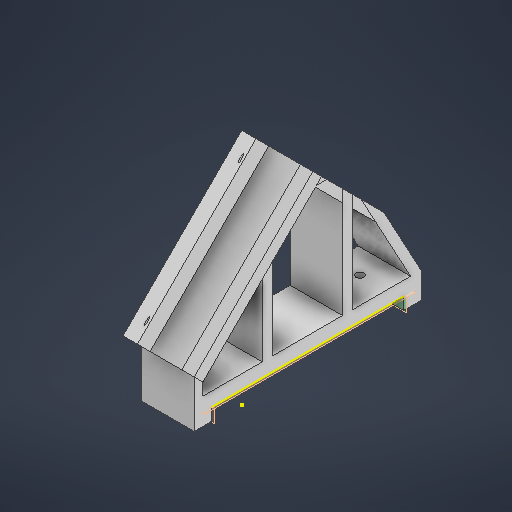
# Autodesk Inventor part: HalterungIso
Saved by Autodesk Inventor 2026.2 (Build 302298000, 298)
## iProperties
Created: 2025-12-13
Part Number: HalterungIso
Material: Generisch
Document SubType Name: Modeling
Designer: alexa
Density: 1 g/cm^3
Appearance: Vorgabe
Author: alexa
Autodesk Inventor part; units mm, degrees
ref_plane "YZ Plane" through (0, 0, 0) normal (1, 0, 0) x (0, 1, 0)
ref_plane "XZ Plane" through (0, 0, 0) normal (0, 1, 0) x (-1, 0, 0)
ref_plane "XY Plane" through (0, 0, 0) normal (0, 0, 1) x (1, 0, 0)
ref_plane "Arbeitsebene1" through (0, 0, 0) normal (0, 0, 1) x (1, 0, 0)
sketch "Skizze1" plane through (0, 0, 0) normal (0, 0, 1) x (1, 0, 0)
  line L0 (15, 55) -> (-15, 55) projected
  line L1 (-15, 55) -> (-15, -55) projected
  line L2 (-15, -55) -> (15, -55) projected
  line L3 (15, -55) -> (15, 55) projected
  circle A0 centre (0, 45) radius 5 projected
  circle A1 centre (0, -45) radius 5 projected
  line L4 (15, 55) -> (-15, 55) projected
  line L5 (-15, 55) -> (-15, -55) projected
  line L6 (-15, -55) -> (15, -55) projected
  line L7 (15, -55) -> (15, 55) projected
  circle A2 centre (0, 45) radius 5 projected
  circle A3 centre (0, -45) radius 5 projected
  point P0 (0, 0)
ref_plane "Arbeitsebene2" through (0, -55, -5) normal (0, -1, 0) x (-1, 0, 0)
sketch "Skizze2" plane through (0, -55, -5) normal (0, -1, 0) x (-1, 0, 0)
  line L0 (15, 2) -> (-15, 2) projected
  line L1 (-15, 2) -> (-15, -2) projected
  line L2 (-15, -2) -> (-15, -5) projected
  line L3 (15, -5) -> (-15, -5) projected
  line L4 (15, 2) -> (15, -5) projected
  point P0 (0, -5)
extrude "Extrusion1" add sketch "Skizze2" along normal blind 10
sketch "Skizze3" plane through (-15, -55, 0) normal (0, 0, 1) x (1, 0, 0)
  line L0 (0, -10) -> (30, -10) projected
  line L1 (30, 0) -> (30, -10) projected
  line L2 (0, -10) -> (30, -10)
  line L3 (30, -10) -> (30, -5)
  line L4 (30, -5) -> (0, -5)
  line L5 (0, -5) -> (0, -10)
  point P0 (15, 55)
  dimension "d2" = 5
  constraints: 8 end point, 2 parallel, 1 horizontal, 1 midpoint, 1 perpendicular
  measures "d2" distance of L3.end L2.end
ref_plane "Arbeitsebene3" through (0, 55, -5) normal (0, 1, 0) x (1, 0, 0)
sketch "Skizze4" plane through (0, 55, -5) normal (0, 1, 0) x (1, 0, 0)
  line L0 (15, 2) -> (15, -5) projected
  line L1 (15, 2) -> (-15, 2) projected
  line L2 (-15, 2) -> (-15, -5) projected
  line L3 (15, -5) -> (-15, -5) projected
  point P0 (0, -5)
extrude "Extrusion2" add sketch "Skizze4" along normal blind 10
sketch "Skizze5" plane through (-15, 55, 0) normal (0, 0, 1) x (1, 0, 0)
  line L0 (0, 10) -> (30, 10) projected
  line L1 (0, 0) -> (0, 10) projected
  line L2 (30, 10) -> (0, 10)
  line L3 (0, 10) -> (0, 5)
  line L4 (0, 5) -> (30, 5)
  line L5 (30, 5) -> (30, 10)
  point P0 (15, -55)
  dimension "d5" = 5
  constraints: 8 end point, 2 parallel, 1 horizontal, 1 midpoint, 1 perpendicular
  measures "d5" distance of L3.end L2.end
extrude "Extrusion3" add sketch "Skizze3" along normal blind 20
sketch "Skizze6" plane through (15, -55, 0) normal (1, 0, 0) x (0, 0, -1)
  line L0 (7, -10) -> (-20, -10) projected
  line L1 (-20, -10) -> (-15, -5)
  line L2 (0, -5) -> (-20, -5) projected
  line L3 (-20, -10) -> (-12.9289, -10) construction
  line L4 (-20, -5) -> (-20, -10)
  point P0 (0, 55)
  dimension "d8" = 45
  constraints: 6 end point, 1 equal length, 1 horizontal, 1 point on line, 1 vertical
  measures "d8" angle of L3 L1
extrude "Extrusion4" cut sketch "Skizze6" against normal blind 46
sketch "Skizze7" plane through (-15, -60, 15) normal (0, 0.7071068, 0.7071068) x (1, 0, 0)
  line L0 (0, -7.0711) -> (0, 0) projected
  line L1 (0, -7.0711) -> (30, -7.0711) projected
  line L2 (30, 0) -> (30, -7.0711) projected
  line L3 (0, 0) -> (30, 0) projected
  point P0 (15, 53.033)
extrude "Extrusion5" add sketch "Skizze7" along normal blind 166
extrude "Extrusion6" add sketch "Skizze5" along normal blind 166
sketch "Skizze8" plane through (-15, 60, 0) normal (0, -1, 0) x (1, 0, 0)
  line L0 (30, 0) -> (0, 0) projected
  line L1 (30, 0) -> (30, 166) projected
  line L2 (0, 166) -> (30, 166) projected
  line L3 (0, 0) -> (0, 166) projected
  line L4 (0, 0) -> (0, 80)
  line L5 (0, 0) -> (0, 166) projected
  line L6 (0, 80) -> (30, 80)
  line L7 (0, 80) -> (30, 80)
  line L8 (30, 80) -> (30, 88)
  line L9 (30, 88) -> (0, 88)
  line L10 (0, 88) -> (0, 80)
  point P0 (15, 0)
  dimension "d15" = 80
  dimension "d16" = 8
  constraints: 12 end point, 3 point on line, 2 parallel, 2 perpendicular, 1 horizontal
  measures "d15" distance of L0.end L4.end
  measures "d16" distance of L8.end L7.end
extrude "Extrusion7" add sketch "Skizze8" along normal blind 57 contours L6 L3 L9 L1
sketch "Skizze9" plane through (-15, -65, -7) normal (-1, 0, 0) x (0, 0, 1)
  line L0 (27, 0) -> (144.3797, 117.3797) projected
  line L1 (139.3797, 122.3797) -> (144.3797, 117.3797) projected
  line L2 (95, 78) -> (139.3797, 122.3797) projected
  line L3 (95, 125) -> (95, 78) projected
  line L4 (95, 125) -> (173, 125) projected
  line L5 (173, 130) -> (173, 125) projected
  line L6 (0, 130) -> (173, 130) projected
  line L7 (0, 120) -> (0, 130) projected
  line L8 (0, 120) -> (7, 120) projected
  line L9 (7, 120) -> (7, 125) projected
  line L10 (7, 125) -> (87, 125) projected
  line L11 (87, 125) -> (87, 70) projected
  line L12 (22, 5) -> (87, 70) projected
  line L13 (7, 5) -> (22, 5) projected
  line L14 (7, 10) -> (7, 5) projected
  line L15 (7, 10) -> (0, 10) projected
  line L16 (0, 10) -> (0, 0) projected
  line L17 (0, 0) -> (27, 0) projected
  line L18 (95, 125) -> (95, 130)
  line L19 (95, 125) -> (95, 78) projected
  line L20 (95, 78) -> (95, 68)
  point P0 (7, 65)
  constraints: 4 end point, 3 point on line, 1 perpendicular
extrude "Extrusion8" cut sketch "Skizze9" against normal blind 61.5 contours L20 L2 L1 L0 | L18 L6 L5 L4
sketch "Skizze10" plane through (-15, 60, 0) normal (0, -1, 0) x (1, 0, 0)
  line L0 (30, 0) -> (30, 80) projected
  line L1 (0, 0) -> (30, 0)
  line L2 (30, 0) -> (30, 8)
  line L3 (30, 8) -> (0, 8)
  line L4 (0, 8) -> (0, 0)
  point P0 (15, 0)
  dimension "d21" = 8
  constraints: 8 end point, 2 parallel, 1 horizontal, 1 perpendicular, 1 point on line
  measures "d21" distance of L2.end L1.end
extrude "Extrusion9" add sketch "Skizze10" along normal blind 123.5
sketch "Skizze12" plane through (-15, 60, 8) normal (0, 0, 1) x (1, 0, 0)
  line L0 (30, -120) -> (0, -120) projected
  line L1 (30, 0) -> (30, -120) projected
  line L2 (0, 0) -> (30, 0) projected
  line L3 (0, 0) -> (0, -120) projected
  line L4 (15, -60) -> (30, -60)
  line L5 (30, 0) -> (30, -120) projected
  line L6 (30, -60) -> (30, -40)
  line L7 (30, -40) -> (30, -80)
  line L8 (0, 0) -> (0, -120) projected
  line L9 (30, -40) -> (0, -40)
  line L10 (0, -40) -> (0, -34)
  line L11 (0, -34) -> (30, -34)
  line L12 (30, -34) -> (30, -40)
  line L13 (30, -80) -> (0, -80)
  line L14 (0, -80) -> (0, -86)
  line L15 (0, -86) -> (30, -86)
  line L16 (30, -86) -> (30, -80)
  dimension "d26" = 20
  dimension "d27" = 40
  dimension "d28" = 6
  dimension "d29" = 6
  constraints: 22 end point, 4 parallel, 4 point on line, 2 horizontal, 2 perpendicular, 1 midpoint
  measures "d26" distance of L4.end L6.end
  measures "d27" distance of L6.end L7.end
  measures "d28" distance of L9.end L10.end
  measures "d29" distance of L14.end L13.end
extrude "Extrusion11" add sketch "Skizze12" along normal blind 76.5 contours L3 L11 L1 L9
sketch "Skizze13" plane through (-15, -60, 8) normal (0, 0, 1) x (1, 0, 0)
  line L0 (0, 80) -> (0, 40)
  line L1 (0, 80) -> (0, 0) projected
  line L2 (30, 80) -> (30, 0) projected
  line L3 (0, 40) -> (30, 40)
  line L4 (30, 40) -> (30, 34)
  line L5 (30, 34) -> (0, 34)
  line L6 (0, 34) -> (0, 40)
  point P0 (15, 60)
  point P1 (0, 34)
  point P2 (30, 40)
  dimension "d32" = 40
  dimension "d33" = 6
  constraints: 10 end point, 2 parallel, 1 horizontal, 1 midpoint, 1 perpendicular, 1 point on line
  measures "d32" distance of L0.start L0.end
  measures "d33" distance of L3.end L4.end
extrude "Extrusion12" add sketch "Skizze13" along normal blind 49.25
sketch "Skizze31" plane through (0, 0, 0) normal (0, 0, 1) x (1, 0, 0)
  point P0 (0, 0)
sketch "Skizze41" plane through (-15, -65, 20) normal (0, -0.7071068, 0.7071068) x (1, 0, 0)
  line L0 (30, 96.1665) -> (0, 96.1665) projected
  line L1 (0, 0) -> (0, 96.1665) projected
  line L2 (0, 0) -> (30, 0) projected
  line L3 (30, 0) -> (30, 96.1665) projected
  line L4 (0, 96.1665) -> (5, 96.1665)
  line L5 (5, 96.1665) -> (5, 0)
  line L6 (5, 0) -> (0, 0)
  line L7 (0, 0) -> (0, 96.1665)
  line L8 (30, 96.1665) -> (0, 96.1665) projected
  line L9 (30, 96.1665) -> (25, 96.1665)
  line L10 (25, 96.1665) -> (25, 0)
  line L11 (25, 0) -> (30, 0)
  line L12 (30, 0) -> (30, 96.1665)
  point P0 (15, 31.8198)
  dimension "d88" = 5
  dimension "d89" = 5
  constraints: 16 end point, 4 parallel, 2 horizontal, 2 perpendicular, 2 point on line
  measures "d88" distance of L5.end L6.end
  measures "d89" distance of L11.end L10.end
extrude "Extrusion34" add sketch "Skizze41" along normal blind 10 contours L3 L2 L10 L0 | L5 L2 L1 L0
sketch "Skizze42" plane through (-10, -65, 20) normal (0, -0.7071068, -0.7071068) x (-1, 0, 0)
  line L0 (5, 0) -> (0, 0) projected
  line L1 (0, 0) -> (0, -10) projected
  line L2 (5, -10) -> (0, -10) projected
  line L3 (5, 0) -> (5, -10) projected
  line L4 (-20, 0) -> (-25, 0) projected
  line L5 (-25, 0) -> (-25, -10) projected
  line L6 (-20, -10) -> (-25, -10) projected
  line L7 (-20, 0) -> (-20, -10) projected
  line L8 (0, -10) -> (5, -5)
  line L9 (-25, -10) -> (-20, -5)
  point P0 (-10, 60.1041)
  constraints: 4 end point, 2 midpoint, 1 parallel
extrude "Extrusion35" cut sketch "Skizze42" against normal blind 136 contours L3 L2 L8 | L7 L6 L9
sketch "Skizze43" plane through (-15, 3, 88) normal (0, 0.7071068, 0.7071068) x (1, 0, 0)
  line L0 (0, -5) -> (5, -10) projected
  line L1 (5, 0) -> (5, -10) projected
  line L2 (5, 0) -> (0, 0) projected
  line L3 (0, 0) -> (0, -5) projected
  line L4 (25, -5) -> (30, -10) projected
  line L5 (30, 0) -> (30, -10) projected
  line L6 (30, 0) -> (25, 0) projected
  line L7 (25, 0) -> (25, -5) projected
  point P0 (15, 60.1041)
extrude "Extrusion36" add sketch "Skizze43" along normal blind 45
sketch "Skizze48" plane through (-10, -65, 20) normal (0, -0.7071068, -0.7071068) x (-1, 0, 0)
  point P0 (-10, 60.1041)
sketch "Skizze49" plane through (-10, -65, 20) normal (0, -0.7071068, -0.7071068) x (-1, 0, 0)
  line L0 (-20, 0) -> (-20, -5) projected
  line L1 (-20, 0) -> (-25, 0) projected
  line L2 (-25, 0) -> (-25, -10) projected
  line L3 (5, 0) -> (5, -5) projected
  line L4 (5, 0) -> (0, 0) projected
  line L5 (0, 0) -> (0, -10) projected
  line L6 (44.1188, -44.1188) -> (39.1188, -49.1188)
  line L7 (31.6188, -56.6188) -> (26.6188, -61.6188)
  line L8 (-25, -10) -> (-20, -5) projected
  line L9 (0, -10) -> (5, -5) projected
  point P0 (-10, 60.1041)
  constraints: 4 end point
extrude "Extrusion41" [suppressed]
sketch "Skizze50" plane through (-15, 34.8198, 119.8198) normal (0, 0.7071068, 0.7071068) x (1, 0, 0)
  line L0 (25, 0) -> (25, -5) projected
  line L1 (5, -10) -> (5, 0) projected
  line L2 (5, 0) -> (0, 0) projected
  line L3 (0, 0) -> (0, -5) projected
  line L4 (30, -10) -> (30, 0) projected
  line L5 (30, 0) -> (25, 0) projected
  line L6 (-34.1188, -49.1188) -> (-39.1188, -44.1188) projected
  line L7 (-21.6188, -61.6188) -> (-26.6188, -56.6188) projected
  line L8 (25, -5) -> (30, -10) projected
  line L9 (0, -5) -> (5, -10) projected
  point P0 (15, 60.1041)
extrude "Extrusion42" [suppressed]
sketch "Skizze51" plane through (15, 3, 88) normal (0, 0.7071068, -0.7071068) x (-1, 0, 0)
  line L0 (0, 0) -> (5, 0) projected
  line L1 (5, 0) -> (5, 45) projected
  line L2 (0, 45) -> (5, 45) projected
  line L3 (0, 0) -> (0, 45) projected
  line L4 (25, 0) -> (30, 0) projected
  line L5 (30, 0) -> (30, 45) projected
  line L6 (25, 45) -> (30, 45) projected
  line L7 (25, 0) -> (25, 45) projected
  line L8 (5, -96.1665) -> (5, 45) projected
  line L9 (0, 45) -> (5, 45)
  line L10 (5, 45) -> (5, 40)
  line L11 (5, 40) -> (0, 40)
  line L12 (0, 40) -> (0, 45)
  line L13 (25, 45) -> (30, 45) projected
  line L14 (25, 45) -> (30, 45)
  line L15 (30, 45) -> (30, 40)
  line L16 (30, 40) -> (25, 40)
  line L17 (25, 40) -> (25, 45)
  point P0 (15, -64.3467)
  point P1 (25, 40)
  point P2 (0, 40)
  point P3 (5, 40)
  dimension "d109" = 5
  dimension "d110" = 5
  constraints: 16 end point, 4 parallel, 2 horizontal, 2 perpendicular, 2 point on line
  measures "d109" distance of L9.end L10.end
  measures "d110" distance of L14.end L15.end
extrude "Extrusion43" add sketch "Skizze51" along normal blind 10 contours L3 L2 L1 L11 | L7 L6 L5 L16
sketch "Skizze52" plane through (15, -65, 20) normal (1, 0, 0) x (0, 0.7071068, -0.7071068)
  line L0 (0, 0) -> (0, 96.1665) projected
  line L1 (0, 96.1665) -> (0, 136.1665) projected
  line L2 (0, 136.1665) -> (10, 136.1665) projected
  line L3 (10, 141.1665) -> (10, 136.1665) projected
  line L4 (-10, 141.1665) -> (10, 141.1665) projected
  line L5 (-10, 0) -> (-10, 96.1665) projected
  line L6 (0, 0) -> (-10, 0) projected
  line L7 (-5, 141.1665) -> (10, 141.1665) projected
  line L8 (10, 141.1665) -> (5, 136.1665)
  line L9 (-10, 96.1665) -> (-10, 141.1665) projected
  point P0 (60.1041, 31.8198)
  constraints: 2 end point, 1 midpoint
extrude "Extrusion44" cut sketch "Skizze52" against normal blind 46.25 contours L8 L3 L2
sketch "Skizze53" plane through (15, 34.8198, 112.7487) normal (0, 0, -1) x (-1, 0, 0)
  line L0 (5, 7.0711) -> (5, 0) projected
  line L1 (5, 7.0711) -> (0, 7.0711) projected
  line L2 (0, 0) -> (0, 7.0711) projected
  line L3 (5, 0) -> (0, 0) projected
  line L4 (25, 0) -> (25, 7.0711) projected
  line L5 (30, 0) -> (25, 0) projected
  line L6 (30, 7.0711) -> (30, 0) projected
  line L7 (30, 7.0711) -> (25, 7.0711) projected
  point P0 (15, -34.8198)
extrude "Extrusion45" add sketch "Skizze53" along normal blind 29.25
sketch "Skizze55" plane through (10, 34.8198, 112.7487) normal (0, -1, 0) x (1, 0, 0)
  line L0 (-20, -24.7487) -> (-25, -24.7487) projected
  line L1 (-20, 0) -> (-20, -24.7487) projected
  line L2 (-25, 0) -> (-20, 0) projected
  line L3 (-25, 0) -> (-25, -24.7487) projected
  line L4 (5, -24.7487) -> (0, -24.7487) projected
  line L5 (5, 0) -> (5, -24.7487) projected
  line L6 (0, 0) -> (5, 0) projected
  line L7 (0, 0) -> (0, -24.7487) projected
  line L8 (5, 0) -> (5, -24.7487) projected
  line L9 (0, 0) -> (0, -24.7487) projected
  line L10 (5, -12.3744) -> (0, -12.3744)
  line L11 (0, -12.3744) -> (0, -7.3744)
  line L12 (0, -7.3744) -> (5, -7.3744)
  line L13 (5, -7.3744) -> (5, -12.3744)
  line L14 (-20, 0) -> (-20, -24.7487) projected
  line L15 (-25, 0) -> (-25, -24.7487) projected
  line L16 (-20, -12.3744) -> (-25, -12.3744)
  line L17 (-25, -12.3744) -> (-25, -17.3744)
  line L18 (-25, -17.3744) -> (-20, -17.3744)
  line L19 (-20, -17.3744) -> (-20, -12.3744)
  line L20 (5, -12.3744) -> (0, -12.3744)
  line L21 (0, -12.3744) -> (0, -17.3744)
  line L22 (0, -17.3744) -> (5, -17.3744)
  line L23 (5, -17.3744) -> (5, -12.3744)
  point P0 (-10, -112.7487)
  point P1 (0, -17.3744)
  point P2 (5, -17.3744)
  point P3 (5, -12.3744)
  point P4 (0, -12.3744)
  point P5 (-25, -17.3744)
  point P6 (-20, -17.3744)
  point P7 (-20, -12.3744)
  point P8 (-25, -12.3744)
  dimension "d124" = 5
  dimension "d125" = 5
  constraints: 24 end point, 6 parallel, 3 horizontal, 3 perpendicular, 3 point on line, 2 midpoint
  measures "d124" distance of L10.end L11.end
  measures "d125" distance of L17.end L16.end
extrude "Extrusion47" add sketch "Skizze55" along normal blind 26 contours L18 L3 L16 L1 | L22 L7 L10 L5
sketch "Skizze57" plane through (10, 34.8198, 88) normal (-1, 0, 0) x (0, 0, 1)
  line L0 (24.7487, 0) -> (12.3744, 0) projected
  line L1 (28.2843, -3.5355) -> (24.7487, 0) projected
  line L2 (12.3744, -19.4454) -> (28.2843, -3.5355) projected
  line L3 (12.3744, 0) -> (12.3744, -19.4454) projected
  line L4 (7.3744, 0) -> (7.3744, -24.4454) projected
  line L5 (0, -31.8198) -> (7.3744, -24.4454) projected
  line L6 (-68, -99.8198) -> (0, -31.8198) projected
  line L7 (-68, -99.8198) -> (-64.4645, -103.3553) projected
  line L8 (35.3553, -3.5355) -> (24.7487, 7.0711) projected
  line L9 (24.7487, 7.0711) -> (0, 7.0711) projected
  line L10 (0, 0) -> (0, 7.0711) projected
  line L11 (7.3744, 0) -> (0, 0) projected
  line L12 (35.3553, -3.5355) -> (31.8198, -7.0711)
  line L13 (31.8198, -7.0711) -> (28.2843, -3.5355)
  line L14 (28.2843, -3.5355) -> (31.8198, 0)
  line L15 (12.3744, 0) -> (7.3744, 0)
  line L16 (7.3744, 0) -> (7.3744, 7.0711)
  line L17 (7.3744, 7.0711) -> (12.3744, 7.0711)
  line L18 (12.3744, 7.0711) -> (12.3744, 0)
  line L19 (-64.4645, -103.3553) -> (3.5355, -35.3553) projected
  line L20 (3.5355, -35.3553) -> (35.3553, -3.5355) projected
  point P0 (-88, -34.8198)
  point P1 (12.3744, 7.0711)
  point P2 (31.8198, -7.0711)
  dimension "d138" = 5
  constraints: 14 end point, 2 parallel, 2 perpendicular, 2 point on line, 1 horizontal
  measures "d138" distance of L8.start L12.end
extrude "Extrusion49" add sketch "Skizze57" along normal blind 23.5
sketch "Skizze73" plane through (15, -65, -7) normal (1, 0, 0) x (0, 0, -1)
  line L0 (-15, 91) -> (-87, 91) projected
  line L1 (-87, 125) -> (-87, 91) projected
  line L2 (-15, 125) -> (-87, 125) projected
  line L3 (-15, 125) -> (-15, 91) projected
  line L4 (-95, 106.8909) -> (-95, 99.8198) projected
  line L5 (-95, 99.8198) -> (-95, 78) projected
  line L6 (-87, 70) -> (-95, 78) projected
  line L7 (-87, 85) -> (-87, 70) projected
  line L8 (-15, 85) -> (-87, 85) projected
  line L9 (-15, 85) -> (-15, 45) projected
  line L10 (-15, 45) -> (-62, 45) projected
  line L11 (-56, 39) -> (-62, 45) projected
  line L12 (-15, 39) -> (-56, 39) projected
  line L13 (-15, 39) -> (-15, 5) projected
  line L14 (-15, 5) -> (-22, 5) projected
  line L15 (-22, 5) -> (-27, 0) projected
  line L16 (0, 0) -> (-27, 0) projected
  line L17 (0, 10) -> (0, 0) projected
  line L18 (0, 10) -> (-7, 10) projected
  line L19 (-7, 120) -> (-7, 10) projected
  line L20 (-7, 120) -> (0, 120) projected
  line L21 (0, 120) -> (0, 130) projected
  line L22 (0, 130) -> (-95, 130) projected
  line L23 (-95, 130) -> (-95, 106.8909) projected
  line L24 (-95, 106.8909) -> (-95, 99.8198) projected
  line L25 (-119.7487, 106.8909) -> (-95, 106.8909) projected
  line L26 (-119.7487, 99.8198) -> (-119.7487, 106.8909) projected
  line L27 (-119.7487, 99.8198) -> (-107.3744, 99.8198) projected
  line L28 (-107.3744, 99.8198) -> (-102.3744, 99.8198) projected
  line L29 (-102.3744, 99.8198) -> (-95, 99.8198) projected
  line L30 (-102.3744, 75.3744) -> (-107.3744, 80.3744) projected
  line L31 (-107.3744, 80.3744) -> (-123.2843, 96.2843) projected
  line L32 (-123.2843, 96.2843) -> (-119.7487, 99.8198) projected
  line L33 (-119.7487, 99.8198) -> (-119.7487, 106.8909) projected
  line L34 (-133.8909, 92.7487) -> (-119.7487, 106.8909) projected
  line L35 (-102.0711, 60.9289) -> (-133.8909, 92.7487) projected
  line L36 (-34.0711, -7.0711) -> (-102.0711, 60.9289) projected
  line L37 (-27, 0) -> (-34.0711, -7.0711) projected
  line L38 (-27, 0) -> (-95, 68) projected
  line L39 (-95, 68) -> (-102.3744, 75.3744) projected
  line L40 (-102.3744, 75.3744) -> (-107.3744, 80.3744) projected
  line L41 (-102.3744, 99.8198) -> (-102.3744, 75.3744) projected
  line L42 (-107.3744, 99.8198) -> (-102.3744, 99.8198) projected
  line L43 (-107.3744, 99.8198) -> (-107.3744, 80.3744) projected
  line L44 (-15, 125) -> (-15, 130)
  line L45 (-87, 125) -> (-87, 91) projected
  line L46 (-87, 91) -> (-109.5711, 68.4289)
  point P0 (-7, 65)
  point P1 (-95, 83)
  point P2 (-102.5, 75.5)
  constraints: 4 end point, 3 point on line, 1 perpendicular
extrude "Extrusion64" cut sketch "Skizze73" against normal blind 119 contours L46 L5 L4 L23 L22 L44 L2 L1 | L29 L28 L27 L26 L25 L4 | L46 L30 L43 L28 L41 | L41 L30 L46 | L46 L35 L34 L26 L32 L31 L30 | L43 L31 L32 L27
sketch "Skizze74" plane through (15, -65, -7) normal (1, 0, 0) x (0, 0, -1)
  line L0 (-15, 91) -> (-87, 91) projected
  line L1 (-15, 91) -> (-15, 130) projected
  line L2 (-87, 91) -> (-15, 130)
  line L3 (-15, 130) -> (-87, 91)
  line L4 (-87, 91) -> (-82, 91)
  line L5 (-15, 130) -> (-15, 124)
  line L6 (-15, 130) -> (-15, 91) projected
  line L7 (-15, 91) -> (-87, 91) projected
  line L8 (-87, 91) -> (-95, 83) projected
  line L9 (-95, 83) -> (-95, 78) projected
  line L10 (-87, 70) -> (-95, 78) projected
  line L11 (-87, 85) -> (-87, 70) projected
  line L12 (-15, 85) -> (-87, 85) projected
  line L13 (-15, 85) -> (-15, 45) projected
  line L14 (-15, 45) -> (-62, 45) projected
  line L15 (-56, 39) -> (-62, 45) projected
  line L16 (-15, 39) -> (-56, 39) projected
  line L17 (-15, 39) -> (-15, 5) projected
  line L18 (-15, 5) -> (-22, 5) projected
  line L19 (-22, 5) -> (-27, 0) projected
  line L20 (0, 0) -> (-27, 0) projected
  line L21 (0, 10) -> (0, 0) projected
  line L22 (0, 10) -> (-7, 10) projected
  line L23 (-7, 120) -> (-7, 10) projected
  line L24 (-7, 120) -> (0, 120) projected
  line L25 (0, 120) -> (0, 130) projected
  line L26 (0, 130) -> (-15, 130) projected
  line L27 (-15, 124) -> (-87, 85)
  point P0 (-7, 65)
  point P1 (-75.9231, 91)
  dimension "d195" = 5
  dimension "d196" = 6
  constraints: 10 end point, 2 point on line, 1 collinear
  measures "d195" distance of L0.end L4.end
  measures "d196" distance of L1.end L5.end
extrude "Extrusion65" add sketch "Skizze74" against normal blind 30 contours L0 L2 L1 L27
sketch "Skizze75" plane through (-15, -65, -7) normal (-1, 0, 0) x (0, 0, 1)
  line L0 (15, 91) -> (75.9231, 91) projected
  line L1 (15, 91) -> (15, 124) projected
  line L2 (15, 124) -> (75.9231, 91) projected
  line L3 (87, 91) -> (15, 130) projected
  line L4 (0, 130) -> (15, 130) projected
  line L5 (0, 120) -> (0, 130) projected
  line L6 (0, 120) -> (7, 120) projected
  line L7 (7, 120) -> (7, 10) projected
  line L8 (7, 10) -> (0, 10) projected
  line L9 (0, 10) -> (0, 0) projected
  line L10 (0, 0) -> (27, 0) projected
  line L11 (27, 0) -> (30.5355, -3.5355) projected
  line L12 (30.5355, -3.5355) -> (106.0355, 71.9645) projected
  line L13 (106.0355, 71.9645) -> (102.5, 75.5) projected
  line L14 (95, 68) -> (102.5, 75.5) projected
  line L15 (95, 68) -> (95, 83) projected
  line L16 (95, 83) -> (87, 91) projected
  line L17 (15, 85) -> (15, 45) projected
  line L18 (15, 85) -> (87, 85) projected
  line L19 (87, 85) -> (87, 70) projected
  line L20 (62, 45) -> (87, 70) projected
  line L21 (15, 45) -> (62, 45) projected
  line L22 (15, 39) -> (56, 39) projected
  line L23 (22, 5) -> (56, 39) projected
  line L24 (15, 5) -> (22, 5) projected
  line L25 (15, 39) -> (15, 5) projected
  line L26 (109.5711, 68.4289) -> (106.0355, 71.9645) projected
  line L27 (30.5355, -3.5355) -> (106.0355, 71.9645) projected
  line L28 (34.0711, -7.0711) -> (30.5355, -3.5355) projected
  line L29 (34.0711, -7.0711) -> (109.5711, 68.4289) projected
  line L30 (95, 68) -> (102.0711, 60.9289)
  point P0 (7, 65)
  constraints: 2 end point, 1 perpendicular, 1 point on line
extrude "Extrusion66" cut sketch "Skizze75" against normal blind 98.25 contours L14 L13 L12 L30 | L12 L26 L29 L30
sketch "Skizze76" plane through (-15, 3, 88) normal (0, 0.7071068, 0.7071068) x (1, 0, 0)
  line L0 (0, 36.0624) -> (0, 12.0208) projected
  line L1 (30, 0) -> (0, 0) projected
  line L2 (5, -10) -> (0, -5) projected
  line L3 (5, -5) -> (5, -10) projected
  line L4 (25, -5) -> (5, -5) projected
  line L5 (25, -5) -> (30, -10) projected
  line L6 (30, 0) -> (30, -10) projected
  line L7 (30, 0) -> (0, 0) projected
  line L8 (0, -5) -> (0, 0) projected
  line L9 (5, -10) -> (25, -30)
  line L10 (30, -10) -> (25, -5)
  line L11 (25, -5) -> (12.5, -17.5)
  line L12 (12.5, -17.5) -> (17.5, -22.5)
  line L13 (17.5, -22.5) -> (30, -10)
  line L14 (17.5, -22.5) -> (28.1066, -33.1066)
  line L15 (28.1066, -33.1066) -> (23.864, -37.3492)
  line L16 (0, -5) -> (28.1066, -33.1066)
  line L17 (28.1066, -33.1066) -> (23.864, -37.3492)
  line L18 (23.864, -37.3492) -> (-4.2426, -9.2426)
  line L19 (-4.2426, -9.2426) -> (0, -5)
  point P0 (15, 60.1041)
  point P1 (17.5, -22.5)
  point P2 (12.5, -17.5)
  point P3 (25, -30)
  dimension "d201" = 15
  dimension "d202" = 6
  constraints: 22 end point, 4 parallel, 3 perpendicular, 2 point on line, 1 collinear
  measures "d201" distance of L12.end L14.end
  measures "d202" distance of L14.end L15.end
extrude "Extrusion67" add sketch "Skizze76" along normal blind 96.25 from surface at -96.1665 contours L13 L9 L11 L5 | L2 L9 L14 L15 L18 L19
sketch "Skizze77" plane through (15, -65, 20) normal (1, 0, 0) x (0, 0.7071068, -0.7071068)
  line L0 (0, 96.1665) -> (-10, 96.1665) projected
  line L1 (-10, 0) -> (-10, 96.1665) projected
  line L2 (0, 0) -> (-10, 0) projected
  line L3 (0, 0) -> (0, 96.1665) projected
  line L4 (-10, 96.1665) -> (-38.8061, 96.1665)
  line L5 (-38.8061, 96.1665) -> (-38.8061, 98.6326)
  line L6 (-38.8061, 98.6326) -> (-10, 98.6326)
  line L7 (-10, 98.6326) -> (-10, 96.1665)
  line L8 (-10, 98.6326) -> (0, 98.6326)
  line L9 (0, 98.6326) -> (0, 96.1665)
  point P0 (60.1041, 31.8198)
  constraints: 12 end point, 3 perpendicular, 2 horizontal
extrude "Extrusion68" cut sketch "Skizze77" against normal blind 125.75 contours L0 L7 L8 L9 | L4 L5 L6 L7
sketch "Skizze78" plane through (13.1066, -20.4099, 111.4099) normal (0.7071068, 0.5, -0.5) x (0, -0.7071068, -0.7071068)
  line L0 (0, 15) -> (0, 0) projected
  line L1 (96.1665, 0) -> (0, 0) projected
  line L2 (96.1665, 0) -> (96.1665, 15) projected
  line L3 (96.1665, 15) -> (0, 15) projected
  line L4 (0, 7.5) -> (15, 7.5)
  circle A0 centre (15, 7.5) radius 2.15
  line L5 (96.1665, 7.5) -> (81.1665, 7.5)
  circle A1 centre (81.1665, 7.5) radius 2.15
  line L6 (15, 7.5) -> (30, 7.5)
  circle A2 centre (30, 7.5) radius 2.15
  line L7 (0, 7.5) -> (10, 7.5)
  line L8 (96.1665, 7.5) -> (86.1665, 7.5)
  circle A3 centre (86.1665, 7.5) radius 2.15
  circle A4 centre (10, 7.5) radius 2.15
  point P0 (64.3467, 75.1777)
  dimension "d207" = 15
  dimension "d208" = 4.3
  dimension "d209" = 15
  dimension "d210" = 4.3
  dimension "d218" = 15
  dimension "d219" = 4.3
  dimension "d224" = 10
  dimension "d225" = 10
  dimension "d226" = 4.3
  constraints: 10 end point, 5 centre point, 5 coincident, 3 horizontal, 2 midpoint, 2 point on line
  measures "d207" distance of L4.start L4.end
  measures "d208" diameter of A0
  measures "d209" distance of L5.start L5.end
  measures "d210" diameter of A1
  measures "d218" distance of L6.start L6.end
  measures "d219" diameter of A2
  measures "d224" distance of L4.start L7.end
  measures "d225" distance of L5.start L8.end
  measures "d226" diameter of A4
extrude "Extrusion69" cut sketch "Skizze78" against normal blind 125.75 contours L4 A4 | L4 A4 | A3 L5 | L5 A3
sketch "Skizze79" plane through (15, -65, 20) normal (1, 0, 0) x (0, 0.7071068, -0.7071068)
  line L0 (7.0711, 91.9239) -> (7.0711, 103.2376) projected
  line L1 (7.0711, 103.2376) -> (0, 96.1665) projected
  line L2 (0, 0) -> (0, 96.1665) projected
  line L3 (7.0711, 0) -> (0, 0) projected
  line L4 (7.0711, 0) -> (7.0711, 48.0833) projected
  line L5 (7.0711, 48.0833) -> (7.0711, 56.5685) projected
  line L6 (7.0711, 56.5685) -> (7.0711, 91.9239) projected
  line L7 (-5, 0) -> (-5, 96.1665) projected
  line L8 (72.832, 55.8614) -> (29.7529, 98.9406) projected
  line L9 (29.7529, 98.9406) -> (96.1665, 79.196) projected
  line L10 (96.1665, 79.196) -> (72.832, 55.8614) projected
  line L11 (68.5894, 51.6188) -> (17.6777, 102.5305) projected
  line L12 (68.5894, 51.6188) -> (40.3051, 23.3345) projected
  line L13 (40.3051, 23.3345) -> (7.0711, 56.5685) projected
  line L14 (7.0711, 48.0833) -> (7.0711, 56.5685) projected
  line L15 (36.0624, 19.0919) -> (7.0711, 48.0833) projected
  line L16 (36.0624, 19.0919) -> (12.0208, -4.9497) projected
  line L17 (12.0208, -4.9497) -> (7.0711, 0) projected
  line L18 (7.0711, 0) -> (0, 0) projected
  line L19 (19.0919, -19.0919) -> (0, 0) projected
  line L20 (26.163, -12.0208) -> (19.0919, -19.0919) projected
  line L21 (26.163, -12.0208) -> (21.2132, -7.0711) projected
  line L22 (98.9949, 70.7107) -> (21.2132, -7.0711) projected
  line L23 (98.9949, 70.7107) -> (103.9447, 65.7609) projected
  line L24 (103.9447, 65.7609) -> (111.0158, 72.832) projected
  line L25 (111.0158, 72.832) -> (100.4092, 83.4386) projected
  line L26 (100.4092, 83.4386) -> (21.9203, 106.7731) projected
  line L27 (21.9203, 106.7731) -> (10.6066, 106.7731) projected
  line L28 (10.6066, 106.7731) -> (7.0711, 103.2376) projected
  line L29 (7.0711, 91.9239) -> (7.0711, 103.2376) projected
  line L30 (17.6777, 102.5305) -> (7.0711, 91.9239) projected
  line L31 (0, 96.1665) -> (89.9839, 96.1665)
  line L32 (89.9839, 96.1665) -> (89.9839, 110.1676)
  line L33 (89.9839, 110.1676) -> (0, 110.1676)
  line L34 (0, 110.1676) -> (0, 96.1665)
  point P0 (60.1041, 31.8198)
  constraints: 8 end point, 3 perpendicular, 1 horizontal
extrude "Extrusion70" cut sketch "Skizze79" against normal blind 125.75 contours L31 L1 L0 | L0 L28 L27 L26 L31 L9 L8 L11 L30 | L30 L11 L31 | L1 L34 L33 L32 L31 L26 L27 L28 | L8 L9 L31
sketch "Skizze80" plane through (15, -60, 15) normal (1, 0, 0) x (0, 0.7071068, -0.7071068)
  line L0 (0, 96.1665) -> (-7.0711, 96.1665) projected
  line L1 (-7.0711, 0) -> (-7.0711, 96.1665) projected
  line L2 (0, 0) -> (-7.0711, 0) projected
  line L3 (0, 0) -> (0, 48.0833) projected
  line L4 (0, 48.0833) -> (0, 56.5685) projected
  line L5 (0, 56.5685) -> (0, 91.9239) projected
  line L6 (0, 91.9239) -> (0, 96.1665) projected
  line L7 (25.4558, 96.1665) -> (16.9706, 96.1665) projected
  line L8 (61.5183, 51.6188) -> (16.9706, 96.1665) projected
  line L9 (61.5183, 51.6188) -> (33.234, 23.3345) projected
  line L10 (33.234, 23.3345) -> (0, 56.5685) projected
  line L11 (0, 48.0833) -> (0, 56.5685) projected
  line L12 (28.9914, 19.0919) -> (0, 48.0833) projected
  line L13 (28.9914, 19.0919) -> (4.9497, -4.9497) projected
  line L14 (4.9497, -4.9497) -> (0, 0) projected
  line L15 (0, 0) -> (-7.0711, 0) projected
  line L16 (12.0208, -19.0919) -> (-7.0711, 0) projected
  line L17 (19.0919, -12.0208) -> (12.0208, -19.0919) projected
  line L18 (19.0919, -12.0208) -> (14.1421, -7.0711) projected
  line L19 (91.9239, 70.7107) -> (14.1421, -7.0711) projected
  line L20 (91.9239, 70.7107) -> (96.8736, 65.7609) projected
  line L21 (96.8736, 65.7609) -> (103.9447, 72.832) projected
  line L22 (103.9447, 72.832) -> (93.3381, 83.4386) projected
  line L23 (93.3381, 83.4386) -> (50.526, 96.1665) projected
  line L24 (50.526, 96.1665) -> (32.0127, 96.1665) projected
  line L25 (32.0127, 96.1665) -> (89.0955, 79.196) projected
  line L26 (89.0955, 79.196) -> (65.7609, 55.8614) projected
  line L27 (65.7609, 55.8614) -> (25.4558, 96.1665) projected
  line L28 (4.2426, 96.1665) -> (0, 96.1665) projected
  line L29 (0, 91.9239) -> (0, 96.1665) projected
  line L30 (4.2426, 96.1665) -> (0, 91.9239) projected
  line L31 (0, 96.1665) -> (0, 91.1665)
  line L32 (0, 91.1665) -> (50.526, 91.1665)
  line L33 (50.526, 91.1665) -> (50.526, 96.1665)
  line L34 (50.526, 96.1665) -> (0, 96.1665)
  point P0 (53.033, 31.8198)
  point P1 (32.0127, 96.1665)
  point P2 (25.4558, 96.1665)
  point P3 (16.9706, 96.1665)
  point P4 (4.2426, 96.1665)
  point P5 (0, 96.1665)
  dimension "d215" = 5
  constraints: 8 end point, 2 parallel, 2 point on line, 1 perpendicular
  measures "d215" distance of L28.end L31.end
extrude "Extrusion71" add sketch "Skizze80" against normal blind 30 contours L28 L30 L6 | L30 L34 L8 L32 L5 | L7 L27 L32 L8 | L34 L25 L32 L27 | L24 L33 L32 L25
sketch "Skizze81" plane through (15, 55, 0) normal (0, 0, -1) x (-1, 0, 0)
  circle A0 centre (15, -10) radius 2.25
  circle A1 centre (15, -100) radius 2.25
  point P0 (15, -55)
  dimension "d220" = 4.5
  dimension "d221" = 4.5
  constraints: 2 centre point, 2 coincident
  measures "d220" diameter of A0
  measures "d221" diameter of A1
extrude "Extrusion72" cut sketch "Skizze81" against normal blind 24.5
sketch "Skizze82" plane through (-15, 43.7273, 47.2727) normal (0, 0.7071068, 0.7071068) x (1, 0, 0)
  line L0 (-4.2426, -66.8397) -> (0, -62.5971) projected
  line L1 (0, -62.5971) -> (0, -46.2834) projected
  line L2 (5, -62.5971) -> (5, -67.5971) projected
  line L3 (0, -62.5971) -> (5, -67.5971)
  line L4 (0, -62.5971) -> (5, -67.5971)
  line L5 (5, -67.5971) -> (8.7477, -63.8494)
  line L6 (8.7477, -63.8494) -> (3.7477, -58.8494)
  line L7 (3.7477, -58.8494) -> (0, -62.5971)
  line L8 (3.7477, -58.8494) -> (0, -62.5971)
  line L9 (0, -62.5971) -> (-4.4106, -58.1865)
  line L10 (-4.4106, -58.1865) -> (-0.6629, -54.4388)
  line L11 (-0.6629, -54.4388) -> (3.7477, -58.8494)
  point P0 (15, 2.507)
  point P1 (0, -55.1017)
  dimension "d227" = 5.3
  constraints: 18 end point, 5 equal length, 2 perpendicular
  measures "d227" distance of L5.end L2.end
extrude "Extrusion73" cut sketch "Skizze82" against normal blind 5.3 contours L7 L6 L5 L3 | L1 L11 L7
fillet "Rundung1" radius 2.515 2 edges at (-12.5, -6.0524, 89.5542) (-11.2523, -1.6346, 85.1365)
